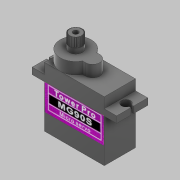
# Autodesk Inventor part: MG90S
Saved by Autodesk Inventor 2022.2 (Build 262287010, 287A)
## iProperties
Created: 2021-05-07
Part Number: MG90S
Material: Resina termoplástica
Document SubType Name: Modeling
Designer: Carlos
Density: 1.28 g/cm^3
Appearance: Suave - Negro
Author: Carlos
Autodesk Inventor part; units mm, degrees
ref_plane "YZ Plane" through (0, 0, 0) normal (1, 0, 0) x (0, 1, 0)
ref_plane "XZ Plane" through (0, 0, 0) normal (0, 1, 0) x (-1, 0, 0)
ref_plane "XY Plane" through (0, 0, 0) normal (0, 0, 1) x (1, 0, 0)
sketch "Boceto1" plane through (0, 0, 0) normal (0, 1, 0) x (-1, 0, 0)
  line L0 (11.5, -6) -> (-11.5, -6)
  line L1 (-11.5, -6) -> (-11.5, 6)
  line L2 (-11.5, 6) -> (11.5, 6)
  line L3 (11.5, 6) -> (11.5, -6)
  line L4 (11.5, -6) -> (-11.5, 6) construction
  line L5 (-11.5, -6) -> (11.5, 6) construction
  point P0 (0, 0)
  dimension "d0" = 23
  dimension "d1" = 12
  constraints: 12 end point, 2 midpoint, 2 parallel, 1 horizontal, 1 perpendicular
  measures "d0" distance of L0.start L0.end
  measures "d1" distance of L0.end L1.end
extrude "Extrusión1" add sketch "Boceto1" along normal blind 23
sketch "Boceto2" plane through (0, 23, 0) normal (0, 1, 0) x (1, 0, 0)
  line L0 (-11.5, -6) -> (11.5, -6) projected
  line L1 (-11.5, 6) -> (-11.5, -6) projected
  line L2 (11.5, 6) -> (-11.5, 6) projected
  arc A0 (-0.1673, 2.75) -> (-0.1673, -2.75) centre (-5.5, 0) ccw
  line L3 (-0.1673, -2.75) -> (1, -2.75)
  line L4 (-0.1673, 2.75) -> (1, 2.75)
  arc A1 (1, -2.75) -> (1, 2.75) centre (1, 0) ccw
  point P0 (0, 0)
  dimension "d5" = 6.5
  constraints: 5 tangent, 4 end point, 4 point on circle, 2 centre point, 2 horizontal
  measures "d5" distance of A1.centre A0.centre
extrude "Extrusión2" add sketch "Boceto2" along normal blind 4.5 contours A0 L4 A1 L3
sketch "Boceto3" plane through (0, 27.5, 0) normal (0, 1, 0) x (1, 0, 0)
  arc A0 (-0.1673, 2.75) -> (-0.1673, -2.75) centre (-5.5, 0) ccw projected
  circle A1 centre (-5.5, 0) radius 2.5
  point P0 (0, 0)
  dimension "d8" = 5
  constraints: 1 centre point, 1 coincident
  measures "d8" diameter of A1
extrude "Extrusión3" add sketch "Boceto3" along normal blind 5.5
sketch "Boceto4" plane through (-5.5, 33, 0) normal (0, 1, 0) x (1, 0, 0)
  line L0 (-0.1459, 2.5797) -> (0, 2.1927)
  line L1 (0, 2.1927) -> (0.1459, 2.5797)
  line L2 (0, 0) -> (0, 0.581) construction
  line L3 (-0.1459, 2.5797) -> (0.1459, 2.5797)
  point P0 (5.5, 0)
  constraints: 8 end point, 1 horizontal, 1 symmetric about line, 1 vertical
extrude "Extrusión4" cut sketch "Boceto4" against normal blind 3.5
pattern_circular "Patrón circular1" count 69 over 360 about axis through (-5.5, 27.5, 0) along (0, -1, 0) of "Extrusión4"
sketch "Boceto5" plane through (0, 33, 0) normal (0, 1, 0) x (1, 0, 0)
  line L0 (-5.6136, 2.4941) -> (-5.6994, 2.1836) projected
  line L1 (-5.6994, 2.1836) -> (-5.84, 2.4734) projected
  line L2 (-5.84, 2.4734) -> (-5.8971, 2.1564) projected
  line L3 (-5.8971, 2.1564) -> (-6.0635, 2.4322) projected
  line L4 (-6.0635, 2.4322) -> (-6.0916, 2.1114) projected
  line L5 (-6.0916, 2.1114) -> (-6.2823, 2.3709) projected
  line L6 (-6.2823, 2.3709) -> (-6.2811, 2.0488) projected
  line L7 (-6.2811, 2.0488) -> (-6.4947, 2.2899) projected
  line L8 (-6.4947, 2.2899) -> (-6.4642, 1.9693) projected
  line L9 (-6.4642, 1.9693) -> (-6.6988, 2.19) projected
  line L10 (-6.6988, 2.19) -> (-6.6393, 1.8735) projected
  line L11 (-6.6393, 1.8735) -> (-6.893, 2.0719) projected
  line L12 (-6.893, 2.0719) -> (-6.8049, 1.7621) projected
  line L13 (-6.8049, 1.7621) -> (-7.0756, 1.9367) projected
  line L14 (-7.0756, 1.9367) -> (-6.9598, 1.6362) projected
  line L15 (-6.9598, 1.6362) -> (-7.2452, 1.7854) projected
  line L16 (-7.2452, 1.7854) -> (-7.1025, 1.4966) projected
  line L17 (-7.1025, 1.4966) -> (-7.4003, 1.6193) projected
  line L18 (-7.4003, 1.6193) -> (-7.232, 1.3447) projected
  line L19 (-7.232, 1.3447) -> (-7.5397, 1.4398) projected
  line L20 (-7.5397, 1.4398) -> (-7.3471, 1.1816) projected
  line L21 (-7.3471, 1.1816) -> (-7.6622, 1.2483) projected
  line L22 (-7.6622, 1.2483) -> (-7.4469, 1.0088) projected
  line L23 (-7.4469, 1.0088) -> (-7.7667, 1.0465) projected
  line L24 (-7.7667, 1.0465) -> (-7.5305, 0.8276) projected
  line L25 (-7.5305, 0.8276) -> (-7.8525, 0.8361) projected
  line L26 (-7.8525, 0.8361) -> (-7.5974, 0.6395) projected
  line L27 (-7.5974, 0.6395) -> (-7.9188, 0.6187) projected
  line L28 (-7.9188, 0.6187) -> (-7.6468, 0.4461) projected
  line L29 (-7.6468, 0.4461) -> (-7.965, 0.3962) projected
  line L30 (-7.965, 0.3962) -> (-7.6785, 0.249) projected
  line L31 (-7.6785, 0.249) -> (-7.9908, 0.1704) projected
  line L32 (-7.9908, 0.1704) -> (-7.6921, 0.0499) projected
  line L33 (-7.6921, 0.0499) -> (-7.996, -0.0568) projected
  line L34 (-7.996, -0.0568) -> (-7.6876, -0.1496) projected
  line L35 (-7.6876, -0.1496) -> (-7.9805, -0.2836) projected
  line L36 (-7.9805, -0.2836) -> (-7.6649, -0.3479) projected
  line L37 (-7.6649, -0.3479) -> (-7.9444, -0.508) projected
  line L38 (-7.9444, -0.508) -> (-7.6243, -0.5434) projected
  line L39 (-7.6243, -0.5434) -> (-7.8881, -0.7281) projected
  line L40 (-7.8881, -0.7281) -> (-7.5661, -0.7343) projected
  line L41 (-7.5661, -0.7343) -> (-7.812, -0.9423) projected
  line L42 (-7.812, -0.9423) -> (-7.4908, -0.9191) projected
  line L43 (-7.4908, -0.9191) -> (-7.7167, -1.1486) projected
  line L44 (-7.7167, -1.1486) -> (-7.3989, -1.0963) projected
  line L45 (-7.3989, -1.0963) -> (-7.6031, -1.3454) projected
  line L46 (-7.6031, -1.3454) -> (-7.2914, -1.2645) projected
  line L47 (-7.2914, -1.2645) -> (-7.472, -1.5311) projected
  line L48 (-7.472, -1.5311) -> (-7.169, -1.4221) projected
  line L49 (-7.169, -1.4221) -> (-7.3246, -1.7041) projected
  line L50 (-7.3246, -1.7041) -> (-7.0327, -1.568) projected
  line L51 (-7.0327, -1.568) -> (-7.1621, -1.863) projected
  line L52 (-7.1621, -1.863) -> (-6.8838, -1.7009) projected
  line L53 (-6.8838, -1.7009) -> (-6.9858, -2.0064) projected
  line L54 (-6.9858, -2.0064) -> (-6.7234, -1.8197) projected
  line L55 (-6.7234, -1.8197) -> (-6.7972, -2.1332) projected
  line L56 (-6.7972, -2.1332) -> (-6.5528, -1.9234) projected
  line L57 (-6.5528, -1.9234) -> (-6.5979, -2.2423) projected
  line L58 (-6.5979, -2.2423) -> (-6.3736, -2.0112) projected
  line L59 (-6.3736, -2.0112) -> (-6.3894, -2.3328) projected
  line L60 (-6.3894, -2.3328) -> (-6.1871, -2.0823) projected
  line L61 (-6.1871, -2.0823) -> (-6.1736, -2.4041) projected
  line L62 (-6.1736, -2.4041) -> (-5.9949, -2.1361) projected
  line L63 (-5.9949, -2.1361) -> (-5.9522, -2.4554) projected
  line L64 (-5.9522, -2.4554) -> (-5.7986, -2.1723) projected
  line L65 (-5.7986, -2.1723) -> (-5.727, -2.4863) projected
  line L66 (-5.727, -2.4863) -> (-5.5998, -2.1904) projected
  line L67 (-5.5998, -2.1904) -> (-5.5, -2.4966) projected
  line L68 (-5.5, -2.4966) -> (-5.4002, -2.1904) projected
  line L69 (-5.4002, -2.1904) -> (-5.273, -2.4863) projected
  line L70 (-5.273, -2.4863) -> (-5.2014, -2.1723) projected
  line L71 (-5.2014, -2.1723) -> (-5.0478, -2.4554) projected
  line L72 (-5.0478, -2.4554) -> (-5.0051, -2.1361) projected
  line L73 (-5.0051, -2.1361) -> (-4.8264, -2.4041) projected
  line L74 (-4.8264, -2.4041) -> (-4.8129, -2.0823) projected
  line L75 (-4.8129, -2.0823) -> (-4.6106, -2.3328) projected
  line L76 (-4.6106, -2.3328) -> (-4.6264, -2.0112) projected
  line L77 (-4.6264, -2.0112) -> (-4.4021, -2.2423) projected
  line L78 (-4.4021, -2.2423) -> (-4.4472, -1.9234) projected
  line L79 (-4.4472, -1.9234) -> (-4.2028, -2.1332) projected
  line L80 (-4.2028, -2.1332) -> (-4.2766, -1.8197) projected
  line L81 (-4.2766, -1.8197) -> (-4.0142, -2.0064) projected
  line L82 (-4.0142, -2.0064) -> (-4.1162, -1.7009) projected
  line L83 (-4.1162, -1.7009) -> (-3.8379, -1.863) projected
  line L84 (-3.8379, -1.863) -> (-3.9673, -1.568) projected
  line L85 (-3.9673, -1.568) -> (-3.6754, -1.7041) projected
  line L86 (-3.6754, -1.7041) -> (-3.831, -1.4221) projected
  line L87 (-3.831, -1.4221) -> (-3.528, -1.5311) projected
  line L88 (-3.528, -1.5311) -> (-3.7086, -1.2645) projected
  line L89 (-3.7086, -1.2645) -> (-3.3969, -1.3454) projected
  line L90 (-3.3969, -1.3454) -> (-3.6011, -1.0963) projected
  line L91 (-3.6011, -1.0963) -> (-3.2833, -1.1486) projected
  line L92 (-3.2833, -1.1486) -> (-3.5092, -0.9191) projected
  line L93 (-3.5092, -0.9191) -> (-3.188, -0.9423) projected
  line L94 (-3.188, -0.9423) -> (-3.4339, -0.7343) projected
  line L95 (-3.4339, -0.7343) -> (-3.1119, -0.7281) projected
  line L96 (-3.1119, -0.7281) -> (-3.3757, -0.5434) projected
  line L97 (-3.3757, -0.5434) -> (-3.0556, -0.508) projected
  line L98 (-3.0556, -0.508) -> (-3.3351, -0.3479) projected
  line L99 (-3.3351, -0.3479) -> (-3.0195, -0.2836) projected
  line L100 (-3.0195, -0.2836) -> (-3.3124, -0.1496) projected
  line L101 (-3.3124, -0.1496) -> (-3.004, -0.0568) projected
  line L102 (-3.004, -0.0568) -> (-3.3079, 0.0499) projected
  line L103 (-3.3079, 0.0499) -> (-3.0092, 0.1704) projected
  line L104 (-3.0092, 0.1704) -> (-3.3215, 0.249) projected
  line L105 (-3.3215, 0.249) -> (-3.035, 0.3962) projected
  line L106 (-3.035, 0.3962) -> (-3.3532, 0.4461) projected
  line L107 (-3.3532, 0.4461) -> (-3.0812, 0.6187) projected
  line L108 (-3.0812, 0.6187) -> (-3.4026, 0.6395) projected
  line L109 (-3.4026, 0.6395) -> (-3.1475, 0.8361) projected
  line L110 (-3.1475, 0.8361) -> (-3.4695, 0.8276) projected
  line L111 (-3.4695, 0.8276) -> (-3.2333, 1.0465) projected
  line L112 (-3.2333, 1.0465) -> (-3.5531, 1.0088) projected
  line L113 (-3.5531, 1.0088) -> (-3.3378, 1.2483) projected
  line L114 (-3.3378, 1.2483) -> (-3.6529, 1.1816) projected
  line L115 (-3.6529, 1.1816) -> (-3.4603, 1.4398) projected
  line L116 (-3.4603, 1.4398) -> (-3.768, 1.3447) projected
  line L117 (-3.768, 1.3447) -> (-3.5997, 1.6193) projected
  line L118 (-3.5997, 1.6193) -> (-3.8975, 1.4966) projected
  line L119 (-3.8975, 1.4966) -> (-3.7548, 1.7854) projected
  line L120 (-3.7548, 1.7854) -> (-4.0402, 1.6362) projected
  line L121 (-4.0402, 1.6362) -> (-3.9244, 1.9367) projected
  line L122 (-3.9244, 1.9367) -> (-4.1951, 1.7621) projected
  line L123 (-4.1951, 1.7621) -> (-4.107, 2.0719) projected
  line L124 (-4.107, 2.0719) -> (-4.3607, 1.8735) projected
  line L125 (-4.3607, 1.8735) -> (-4.3012, 2.19) projected
  line L126 (-4.3012, 2.19) -> (-4.5358, 1.9693) projected
  line L127 (-4.5358, 1.9693) -> (-4.5053, 2.2899) projected
  line L128 (-4.5053, 2.2899) -> (-4.7189, 2.0488) projected
  line L129 (-4.7189, 2.0488) -> (-4.7177, 2.3709) projected
  line L130 (-4.7177, 2.3709) -> (-4.9084, 2.1114) projected
  line L131 (-4.9084, 2.1114) -> (-4.9365, 2.4322) projected
  line L132 (-4.9365, 2.4322) -> (-5.1029, 2.1564) projected
  line L133 (-5.1029, 2.1564) -> (-5.16, 2.4734) projected
  line L134 (-5.16, 2.4734) -> (-5.3006, 2.1836) projected
  line L135 (-5.3006, 2.1836) -> (-5.3864, 2.4941) projected
  line L136 (-5.3864, 2.4941) -> (-5.5, 2.1927) projected
  line L137 (-5.5, 2.1927) -> (-5.6136, 2.4941) projected
  arc A0 (-0.1673, 2.75) -> (-0.1673, -2.75) centre (-5.5, 0) ccw projected
  circle A1 centre (-5.5, 0) radius 1
  point P0 (0, 0)
  dimension "d16" = 2
  constraints: 1 centre point, 1 coincident
  measures "d16" diameter of A1
extrude "Extrusión5" cut sketch "Boceto5" against normal blind 2 contours A1
sketch "Boceto6" plane through (11.5, 0, 6) normal (1, 0, 0) x (0, 0, -1)
  line L0 (0, 0) -> (0, 23) projected
  line L1 (12, 0) -> (12, 23) projected
  line L2 (0, 19) -> (12, 19)
  line L3 (12, 19) -> (12, 16.5)
  line L4 (12, 16.5) -> (0, 16.5)
  line L5 (0, 16.5) -> (0, 19)
  line L6 (0, 0) -> (12, 0) projected
  point P0 (6, 0)
  point P1 (0, 16.5)
  dimension "d19" = 16.5
  dimension "d20" = 2.5
  constraints: 8 end point, 2 parallel, 2 point on line, 1 horizontal, 1 perpendicular
  measures "d19" distance between parallel lines of L4 L6
  measures "d20" distance between parallel lines of L4 L2
extrude "Extrusión6" add sketch "Boceto6" along normal blind 4.75 contours L0 L2 L1 L4
sketch "Boceto7" plane through (-11.5, 0, -6) normal (-1, 0, 0) x (0, 0, 1)
  line L0 (12, 19) -> (0, 19) projected
  line L1 (12, 0) -> (12, 23) projected
  line L2 (0, 19) -> (12, 19)
  line L3 (12, 19) -> (12, 16.5)
  line L4 (12, 16.5) -> (0, 16.5)
  line L5 (0, 16.5) -> (0, 19)
  point P0 (6, 0)
  dimension "d23" = 2.5
  constraints: 8 end point, 2 parallel, 1 horizontal, 1 perpendicular, 1 point on line
  measures "d23" distance between parallel lines of L4 L0
extrude "Extrusión7" add sketch "Boceto7" along normal blind 4.75
sketch "Boceto8" plane through (-11.5, 19, 6) normal (0, 1, 0) x (1, 0, 0)
  circle A0 centre (-2.375, 6) radius 1.75
  circle A1 centre (25.375, 6) radius 1.75
  line L0 (0, 0) -> (-4.75, 0) projected
  line L1 (23, 0) -> (27.75, 0) projected
  line L2 (-4.75, 0) -> (-4.75, 12) projected
  line L3 (27.75, 12) -> (27.75, 0) projected
  point P0 (11.5, 6)
  dimension "d26" = 6
  dimension "d27" = 6
  dimension "d28" = 2.375
  dimension "d29" = 2.375
  dimension "d30" = 3.5
  dimension "d31" = 3.5
  constraints: 2 centre point
  measures "d26" distance from line of L0 A0.centre
  measures "d27" distance from line of L1 A1.centre
  measures "d28" distance from line of L2 A0.centre
  measures "d29" distance from line of L3 A1.centre
  measures "d30" diameter of A0
  measures "d31" diameter of A1
extrude "Extrusión8" cut sketch "Boceto8" against normal up to surface (2.5 mm away)
sketch "Boceto9" plane through (-11.5, 19, 6) normal (0, 1, 0) x (1, 0, 0)
  line L0 (29.4711, 5.5) -> (25.8612, 5.5)
  line L1 (25.8612, 5.5) -> (25.8612, 6.5)
  line L2 (25.8612, 6.5) -> (29.4711, 6.5)
  line L3 (29.4711, 6.5) -> (29.4711, 5.5)
  line L4 (-6.1718, 5.5) -> (-3.3425, 5.5)
  line L5 (-3.3425, 5.5) -> (-3.3425, 6.5)
  line L6 (-3.3425, 6.5) -> (-6.1718, 6.5)
  line L7 (-6.1718, 6.5) -> (-6.1718, 5.5)
  line L8 (0, 0) -> (-4.75, 0) projected
  line L9 (23, 0) -> (27.75, 0) projected
  point P0 (11.5, 6)
  dimension "d34" = 5.5
  dimension "d35" = 5.5
  dimension "d36" = 1
  dimension "d37" = 1
  constraints: 16 end point, 4 parallel, 2 horizontal, 2 perpendicular, 2 point on line
  measures "d34" distance between parallel lines of L4 L8
  measures "d35" distance between parallel lines of L0 L9
  measures "d36" distance of L2.end L0.start
  measures "d37" distance of L6.end L4.start
extrude "Extrusión9" cut sketch "Boceto9" against normal through all
sketch "Boceto10" plane through (-11.5, 0, 6) normal (0, 0, 1) x (1, 0, 0)
  line L0 (0, 0) -> (0, 16.5) projected
  line L1 (0, 16.5) -> (22.8555, 16.7028) construction
  line L2 (22.8555, 16.7028) -> (22.9453, 6.5897) construction
  line L3 (22.9453, 6.5897) -> (0.0897, 6.3869) construction
  line L4 (0.0897, 6.3869) -> (0, 16.5) construction
  point P0 (11.5, 0)
  constraints: 2 other
decal "Calcomanía1"
sketch "Boceto11" plane through (11.5, 0, -6) normal (0, 0, -1) x (-1, 0, 0)
  line L0 (-0.0117, 16.4944) -> (23.0398, 16.4944) construction
  line L1 (23.0398, 16.4944) -> (23.0398, 6.2947) construction
  line L2 (23.0398, 6.2947) -> (-0.0117, 6.2947) construction
  line L3 (-0.0117, 6.2947) -> (-0.0117, 16.4944) construction
  point P0 (11.5, 0)
  constraints: 2 other
decal "Calcomanía2"
